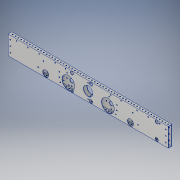
# Autodesk Inventor part: Side Extrusion
Saved by Autodesk Inventor 2019.4 (Build 234330000, 330)
## iProperties
Created: 2019-11-02
Part Number: Side Extrusion
Material: Aluminum 6061
Document SubType Name: Modeling
Designer: admin
Density: 2.7 g/cm^3
Appearance: Aluminum - Flat
Mass: 949.784 g
Surface Area: 3620.83 cm^2
Volume: 351.772 cm^3
Author: admin
Autodesk Inventor part; units mm, degrees
ref_plane "YZ Plane" through (0, 0, 0) normal (1, 0, 0) x (0, 1, 0)
ref_plane "XZ Plane" through (0, 0, 0) normal (0, 1, 0) x (-1, 0, 0)
ref_plane "XY Plane" through (0, 0, 0) normal (0, 0, 1) x (1, 0, 0)
sketch "Sketch1" plane through (0, 0, 0) normal (1, 0, 0) x (0, 1, 0)
  line L0 (-50, 10) -> (50, 10)
  line L1 (50, 10) -> (50, -10)
  line L2 (50, -10) -> (-50, -10)
  line L3 (-50, -10) -> (-50, 10)
  line L4 (-50, 10) -> (50, -10) construction
  line L5 (50, 10) -> (-50, -10) construction
  line L6 (48, -8) -> (48, 8)
  line L7 (48, 8) -> (-48, 8)
  line L8 (-48, 8) -> (-48, -8)
  line L9 (-48, -8) -> (48, -8)
  point P0 (0, 0)
  dimension "d0" = 100
  dimension "d1" = 20
  dimension "d2" = 2
  constraints: 20 end point, 4 parallel, 2 midpoint, 2 perpendicular, 1 horizontal, 3 other
  measures "d0" distance of L1.end L2.end
  measures "d1" distance of L0.end L1.end
  measures "d2" distance between parallel lines of L1 L6
extrude "Extrusion1" add sketch "Sketch1" along normal blind 850
sketch "Sketch2" plane through (0, -50, 10) normal (0, 0, -1) x (-1, 0, 0)
  circle A0 centre (-200, 18.3) radius 16.3
  line L0 (0, 0) -> (-850, 0) projected
  line L1 (0, 100) -> (0, 0) projected
  line L2 (0, 100) -> (-850, 100) projected
  line L3 (0, 0) -> (-850, 0) projected
  circle A1 centre (-650, 18.3) radius 16.3
  line L4 (-850, 100) -> (-850, 0) projected
  point P0 (0, 50)
  dimension "d5" = 32.6
  dimension "d9" = 200
  dimension "d113" = 200
  constraints: 2 centre point
  measures "d5" diameter of A0
  measures "d9" distance from line of L1 A0.centre
  measures "d113" distance from line of L4 A1.centre
extrude "Extrusion2" cut sketch "Sketch2" along normal blind 2 contours A0 | A1
sketch "Sketch3" plane through (0, -50, 10) normal (0, 0, 1) x (1, 0, 0)
  circle A0 centre (320, 36) radius 34
  line L0 (0, 0) -> (0, 100) projected
  line L1 (0, 0) -> (850, 0) projected
  line L2 (425, 100) -> (425, 0)
  circle A1 centre (530, 36) radius 34
  point P0 (0, 50)
  dimension "d10" = 68
  dimension "d11" = 320
  dimension "d12" = 36
  constraints: 2 centre point, 2 end point, 1 midpoint, 1 symmetric about line, 1 other
  measures "d10" diameter of A0
  measures "d11" distance from line of L0 A0.centre
  measures "d12" distance from line of A0.centre L1
extrude "Extrusion3" cut sketch "Sketch3" against normal blind 2
sketch "Sketch4" plane through (0, -50, -10) normal (0, 0, -1) x (-1, 0, 0)
  circle A0 centre (-200, 18.3) radius 16.3 construction
  circle A1 centre (-200, 18.3) radius 16.3 construction
  circle A2 centre (-200, 18.3) radius 12.3
  line L0 (0, 0) -> (-850, 0) projected
  line L1 (-425, 0) -> (-425, 100)
  line L2 (0, 100) -> (-850, 100) projected
  circle A3 centre (-650, 18.3) radius 12.3
  point P0 (0, 50)
  point P1 (-200, 2)
  dimension "d17" = 24.6
  constraints: 2 centre point, 2 end point, 2 midpoint, 1 coincident, 1 symmetric about line, 1 vertical alignment, 1 other
  measures "d17" diameter of A2
extrude "Extrusion4" cut sketch "Sketch4" against normal blind 2
sketch "Sketch5" plane through (0, -50, -10) normal (0, 0, -1) x (-1, 0, 0)
  circle A0 centre (-216, 18.3) radius 2.25
  circle A1 centre (-200, 18.3) radius 12.3 projected
  line L0 (-200, 18.3) -> (-216, 18.3) construction
  circle A2 centre (-200, 34.3) radius 2.25
  circle A3 centre (-184, 18.3) radius 2.25
  line L1 (0, 100) -> (-850, 100) projected
  line L2 (-425, 100) -> (-425, 0)
  line L3 (0, 0) -> (-850, 0) projected
  circle A4 centre (-634, 18.3) radius 2.25
  circle A5 centre (-650, 34.3) radius 2.25
  circle A6 centre (-666, 18.3) radius 2.25
  point P0 (0, 50)
  dimension "d18" = 4.5
  dimension "d21" = 16
  dimension "d24" = 180
  constraints: 6 centre point, 4 end point, 3 symmetric about line, 2 midpoint, 1 horizontal, 8 other
  measures "d18" diameter of A0
  measures "d21" distance of L0.start L0.end
extrude "Extrusion5" cut sketch "Sketch5" against normal blind 2 contours A0 | A2 | A3 | A4 | A5 | A6
sketch "Sketch6" plane through (0, -50, -10) normal (0, 0, -1) x (-1, 0, 0)
  circle A0 centre (-320, 36) radius 10
  line L0 (0, 0) -> (-850, 0)
  line L1 (0, 100) -> (0, 0)
  circle A1 centre (-320, 36) radius 25.4
  circle A2 centre (-320, 61.4) radius 2.75
  circle A3 centre (-345.4, 36) radius 2.75
  circle A4 centre (-320, 10.6) radius 2.75
  circle A5 centre (-294.6, 36) radius 2.75
  line L2 (-253.082685, 23.409359) -> (-232.819395, 42.510891)
  arc A6 (-232.819395, 42.510891) -> (-221.835325, 43.130108) centre (-228.087042, 56.296226) ccw
  line L3 (-221.835325, 43.130108) -> (-214.280231, 31.689157)
  arc A7 (-214.280231, 31.689157) -> (-219.289116, 21.635076) centre (-200.000275, 18.300226) ccw
  line L4 (-219.289116, 21.635076) -> (-250.702863, 18.243714)
  arc A8 (-253.082685, 23.409359) -> (-250.702863, 18.243714) centre (-251.024866, 21.226383) ccw
  line L5 (-211.509077, 53.460841) -> (-194.873767, 53.460841)
  arc A9 (-192.370348, 52.113987) -> (-194.873767, 53.460841) centre (-194.873767, 50.460841) ccw
  line L6 (-192.370348, 52.113987) -> (-179.138449, 32.076445)
  arc A10 (-175.036603, 16.95297) -> (-179.138449, 32.076445) centre (-200.000275, 18.300226) ccw
  arc A11 (-178.032244, 14.114641) -> (-175.036603, 16.95297) centre (-178.032244, 17.114641) ccw
  arc A12 (-180.454865, 17.224322) -> (-178.032244, 14.114641) centre (-177.459399, 17.059432) ccw
  arc A13 (-180.454865, 17.224322) -> (-207.063381, 36.556544) centre (-200.000275, 18.300226) ccw
  arc A14 (-210.571115, 37.588637) -> (-207.063381, 36.556544) centre (-208.145849, 39.354447) ccw
  line L7 (-210.571115, 37.588637) -> (-215.850481, 44.839623)
  arc A15 (-215.927945, 48.259622) -> (-215.850481, 44.839623) centre (-213.425215, 46.605433) ccw
  arc A16 (-215.927945, 48.259622) -> (-214.338886, 51.456924) centre (-228.087042, 56.296226) ccw
  arc A17 (-211.509077, 53.460841) -> (-214.338886, 51.456924) centre (-211.509077, 50.460841) ccw
  line L8 (-284.50186, 40.584929) -> (-284.231798, 32.883294)
  arc A18 (-288.442052, 30.033928) -> (-284.231798, 32.883294) centre (-287.229955, 32.778162) ccw
  line L9 (-288.442052, 30.033928) -> (-290.947932, 31.140747)
  arc A19 (-305.806233, 47.249065) -> (-290.947932, 31.140747) centre (-279.837042, 56.296226) ccw
  arc A20 (-302.97323, 51.236028) -> (-305.806233, 47.249065) centre (-302.97323, 48.236028) ccw
  line L10 (-302.97323, 51.236028) -> (-295.454783, 51.236028)
  arc A21 (-292.788881, 49.61188) -> (-295.454783, 51.236028) centre (-295.454783, 48.236028) ccw
  arc A22 (-292.788881, 49.61188) -> (-286.19197, 43.179614) centre (-279.837042, 56.296226) ccw
  arc A23 (-284.50186, 40.584929) -> (-286.19197, 43.179614) centre (-287.500018, 40.479797) ccw
  arc A24 (-214.732134, -2.522909) -> (-211.723391, 2.623837) centre (-213.520037, 0.221325) ccw
  line L11 (-214.732134, -2.522909) -> (-233.31096, 5.683148)
  arc A25 (-232.524215, 11.397075) -> (-233.31096, 5.683148) centre (-232.098863, 8.427382) ccw
  line L12 (-232.524215, 11.397075) -> (-221.426068, 12.986676)
  arc A26 (-218.209959, 11.117746) -> (-221.426068, 12.986676) centre (-221.000715, 10.016983) ccw
  arc A27 (-218.209959, 11.117746) -> (-211.723391, 2.623837) centre (-200.000275, 18.300226) ccw
  line L13 (-193.453229, -3.079233) -> (-193.473523, -1.544854)
  arc A28 (-192.26411, 0.31878) -> (-193.473523, -1.544854) centre (-191.473698, -1.518405) ccw
  arc A29 (-192.26411, 0.31878) -> (-186.409522, 4.212215) centre (-200.000275, 18.300226) ccw
  arc A30 (-185.020939, 4.772827) -> (-186.409522, 4.212215) centre (-185.020939, 2.772827) ccw
  line L14 (-185.020939, 4.772827) -> (-183.032662, 4.772827)
  arc A31 (-181.557218, 1.422618) -> (-183.032662, 4.772827) centre (-183.032662, 2.772827) ccw
  arc A32 (-190.710198, -4.909567) -> (-181.557218, 1.422618) centre (-200.000275, 18.300226) ccw
  arc A33 (-193.453229, -3.079233) -> (-190.710198, -4.909567) centre (-191.453404, -3.052783) ccw
  line L15 (-284.569395, 79.544037) -> (-284.569395, 72.078853)
  arc A34 (-286.249506, 69.384806) -> (-284.569395, 72.078853) centre (-287.569395, 72.078853) ccw
  arc A35 (-286.249506, 69.384806) -> (-292.788881, 62.980572) centre (-279.837042, 56.296226) ccw
  arc A36 (-295.454783, 61.356424) -> (-292.788881, 62.980572) centre (-295.454783, 64.356424) ccw
  line L16 (-295.454783, 61.356424) -> (-302.97323, 61.356424)
  arc A37 (-305.806233, 65.343387) -> (-302.97323, 61.356424) centre (-302.97323, 64.356424) ccw
  arc A38 (-288.516214, 82.390707) -> (-305.806233, 65.343387) centre (-279.837042, 56.296226) ccw
  arc A39 (-284.569395, 79.544037) -> (-288.516214, 82.390707) centre (-287.569395, 79.544037) ccw
  line L17 (-228.57644, 83.796226) -> (-228.087042, 83.796226)
  arc A40 (-205.139033, 71.450067) -> (-228.087042, 83.796226) centre (-228.087042, 56.296226) ccw
  line L18 (-205.139033, 71.450067) -> (-200.077204, 63.784757)
  arc A41 (-202.580623, 59.131611) -> (-200.077204, 63.784757) centre (-202.580623, 62.131611) ccw
  line L19 (-202.580623, 59.131611) -> (-211.509077, 59.131611)
  arc A42 (-214.338886, 61.135528) -> (-211.509077, 59.131611) centre (-211.509077, 62.131611) ccw
  arc A43 (-214.338886, 61.135528) -> (-226.317651, 70.763426) centre (-228.087042, 56.296226) ccw
  arc A44 (-228.765396, 72.69578) -> (-226.317651, 70.763426) centre (-225.953454, 73.741237) ccw
  line L20 (-228.765396, 72.69578) -> (-231.388383, 79.750769)
  arc A45 (-228.57644, 83.796226) -> (-231.388383, 79.750769) centre (-228.57644, 80.796226) ccw
  line L21 (-265.77495, 52.463707) -> (-242.149133, 52.463707)
  arc A46 (-242.149133, 52.463707) -> (-238.347574, 45.944796) centre (-228.087042, 56.296226) ccw
  line L22 (-238.347574, 45.944796) -> (-267.246983, 24.918347)
  arc A47 (-271.92876, 26.642518) -> (-267.246983, 24.918347) centre (-269.011975, 27.344208) ccw
  line L23 (-271.92876, 26.642518) -> (-275.089001, 39.779003)
  arc A48 (-273.480579, 43.180357) -> (-275.089001, 39.779003) centre (-272.172217, 40.480693) ccw
  arc A49 (-273.480579, 43.180357) -> (-265.77495, 52.463707) centre (-279.837042, 56.296226) ccw
  line L24 (-244.279549, 60.128745) -> (-263.644534, 60.128745)
  arc A50 (-266.408547, 61.962454) -> (-263.644534, 60.128745) centre (-263.644534, 63.128745) ccw
  arc A51 (-266.408547, 61.962454) -> (-271.422142, 68.196649) centre (-279.837042, 56.296226) ccw
  arc A52 (-272.690087, 70.646136) -> (-271.422142, 68.196649) centre (-269.690087, 70.646136) ccw
  line L25 (-272.690087, 70.646136) -> (-272.690087, 80.796226)
  arc A53 (-269.690087, 83.796226) -> (-272.690087, 80.796226) centre (-269.690087, 80.796226) ccw
  line L26 (-269.690087, 83.796226) -> (-241.990418, 83.796226)
  arc A54 (-239.348489, 82.217567) -> (-241.990418, 83.796226) centre (-241.990418, 80.796226) ccw
  line L27 (-239.348489, 82.217567) -> (-234.326691, 72.883258)
  arc A55 (-235.452561, 68.873179) -> (-234.326691, 72.883258) centre (-236.96862, 71.461917) ccw
  arc A56 (-235.452561, 68.873179) -> (-241.515537, 61.962454) centre (-228.087042, 56.296226) ccw
  arc A57 (-244.279549, 60.128745) -> (-241.515537, 61.962454) centre (-244.279549, 63.128745) ccw
  circle A58 centre (-188.087042, 69.219) radius 2.75
  circle A59 centre (-277.837042, 16.582759) radius 2.75
  circle A60 centre (-250.087042, 92.776017) radius 2.75
  circle A61 centre (-160.000305, 27.300362) radius 2.75
  circle A62 centre (-313.422276, 79.81286) radius 2.75
  circle A63 centre (-200.000275, 18.300226) radius 9.575
  circle A64 centre (-228.087042, 56.296226) radius 9.575
  circle A65 centre (-279.837042, 56.296226) radius 9.575
  arc A66 (-244.094047, 93.065872) -> (-256.080036, 92.486162) centre (-250.087042, 92.776017) ccw
  line L28 (-256.080036, 92.486162) -> (-281.527863, 91.255361)
  arc A67 (-281.527863, 91.255361) -> (-302.063851, 83.332663) centre (-279.837042, 56.296226) ccw
  line L29 (-312.063851, 85.657061) -> (-302.063851, 83.332663)
  arc A68 (-312.063851, 85.657061) -> (-318.449419, 76.537524) centre (-313.422276, 79.81286) ccw
  line L30 (-312.844999, 67.935588) -> (-318.449419, 76.537524)
  arc A69 (-312.844999, 67.935588) -> (-294.877776, 24.692804) centre (-279.837042, 56.296226) ccw
  line L31 (-294.877776, 24.692804) -> (-283.254771, 19.16117)
  arc A70 (-283.254771, 19.16117) -> (-272.419312, 14.004347) centre (-277.837042, 16.582759) ccw
  line L32 (-272.419312, 14.004347) -> (-215.041009, -13.303196)
  arc A71 (-169.897664, 36.156116) -> (-170.793719, 37.586933) centre (-200.000275, 18.300226) ccw
  line L33 (-160.000305, 21.300362) -> (-162.000275, 21.300362)
  arc A72 (-160.000305, 21.300362) -> (-156.580779, 22.370166) centre (-160.000305, 27.300362) ccw
  arc A73 (-215.041009, -13.303196) -> (-165.000275, 18.300352) centre (-200.000275, 18.300226) ccw
  line L34 (-170.793719, 37.586933) -> (-184.354376, 58.122326)
  arc A74 (-187.633238, 75.201814) -> (-191.393334, 74.225838) centre (-188.087042, 69.219) ccw
  line L35 (-195.5499, 75.076111) -> (-196.794303, 76.960555)
  arc A75 (-196.794303, 76.960555) -> (-229.898636, 93.752442) centre (-228.087042, 56.296226) ccw
  line L36 (-229.898636, 93.752442) -> (-244.094047, 93.065872)
  line L37 (0, 100) -> (-850, 100)
  line L38 (-425, 100) -> (-425, 0)
  circle A76 centre (-530, 61.4) radius 2.75
  circle A77 centre (-504.6, 36) radius 2.75
  circle A78 centre (-530, 10.6) radius 2.75
  circle A79 centre (-555.4, 36) radius 2.75
  circle A80 centre (-661.912958, 69.219) radius 2.75
  circle A81 centre (-572.162958, 16.582759) radius 2.75
  circle A82 centre (-599.912958, 92.776017) radius 2.75
  circle A83 centre (-689.999695, 27.300362) radius 2.75
  circle A84 centre (-536.577724, 79.81286) radius 2.75
  line L39 (-156.580779, 22.370166) -> (-137.281762, 35.755737)
  arc A85 (-137.281762, 35.755737) -> (-147.167505, 72.132439) centre (-148.680183, 52.189726) ccw
  line L40 (-147.167505, 72.132439) -> (-187.633238, 75.201814)
  arc A86 (-195.5499, 75.076111) -> (-191.393334, 74.225838) centre (-193.046481, 76.729257) ccw
  arc A87 (-162.000275, 21.300362) -> (-165.000275, 18.300352) centre (-162.000275, 18.300362) ccw
  circle A88 centre (-148.680183, 52.189726) radius 10.5
  circle A89 centre (-163.234444, 48.560195) radius 1.65
  arc A90 (-181.624055, 62.766879) -> (-184.354376, 58.122326) centre (-181.850957, 59.775472) ccw
  line L41 (-181.624055, 62.766879) -> (-170.444252, 61.918877)
  arc A91 (-167.802767, 58.048634) -> (-170.444252, 61.918877) centre (-170.671154, 58.92747) ccw
  arc A92 (-167.802767, 58.048634) -> (-164.446092, 39.883788) centre (-148.680183, 52.189726) ccw
  arc A93 (-165.101215, 35.572799) -> (-164.446092, 39.883788) centre (-166.810978, 38.037897) ccw
  line L42 (-165.101215, 35.572799) -> (-165.607677, 35.221523)
  arc A94 (-169.897664, 36.156116) -> (-165.607677, 35.221523) centre (-167.31744, 37.686621) ccw
  circle A95 centre (-144.546319, 66.608851) radius 1.65
  circle A96 centre (-138.259787, 41.400132) radius 1.65
  circle A97 centre (-530, 36) radius 10
  point P0 (0, 50)
  point P1 (-200.000275, 18.300226)
  point P2 (-200.000275, 18.300226)
  dimension "d31" = 50.8
  dimension "d28" = 20
  dimension "d29" = 36
  dimension "d30" = 320
  dimension "d32" = 5.5
  dimension "d35" = 360
  dimension "d46" = 36
  constraints: 15 centre point, 10 symmetric about line, 2 end point, 2 midpoint, 1 coincident, 1 vertical alignment, 21 other
  measures "d28" diameter of A0
  measures "d29" distance from line of L0 A0.centre
  measures "d30" distance from line of L1 A0.centre
  measures "d32" diameter of A2
  measures "d46" distance from line of L0 A3.centre
extrude "Extrusion6" cut sketch "Sketch6" against normal blind 50 contours A0 | A2 A1 | A1 A2 | A4 A1 | A1 A4 | A5 A1 | A1 A5 A19 | A5 A19 | A3 A1 | A1 A3 | A58 | A59 | A60 | A61 | A62 | A76 | A77 | A78 | A79 | A80 | A81 | A82 | A83 | A84 | A97 picked at (-296.100043, 35.292407)
sketch "Sketch7" plane through (0, -50, -10) normal (0, 0, -1) x (-1, 0, 0)
  circle A0 centre (-228.087, 56.296) radius 10.5
  line L0 (0, 100) -> (-850, 100) projected
  line L1 (0, 100) -> (0, 0) projected
  circle A1 centre (-279.787, 56.296) radius 10.5
  line L2 (-228.087, 56.296) -> (-279.787, 56.296) construction
  line L3 (-425, 100) -> (-425, 0)
  circle A2 centre (-621.913, 56.296) radius 10.5
  circle A3 centre (-570.213, 56.296) radius 10.5
  point P0 (0, 50)
  dimension "d39" = 43.704
  dimension "d40" = 228.087
  dimension "d41" = 21
  dimension "d44" = 21
  dimension "d45" = 51.7
  constraints: 4 centre point, 4 end point, 2 symmetric about line, 1 horizontal, 1 midpoint, 1 vertical, 2 other
  measures "d39" distance from line of L0 L2.start
  measures "d40" distance from line of L1 L2.start
  measures "d41" diameter of A0
  measures "d44" diameter of A1
  measures "d45" distance of L2.start L2.end
extrude "Extrusion7" cut sketch "Sketch7" against normal up to surface (2 mm away)
sketch "Sketch8" plane through (0, -50, -10) normal (0, 0, -1) x (-1, 0, 0)
  circle A0 centre (-425, 87.5) radius 2.75
  circle A1 centre (-545, 92) radius 2.75
  circle A2 centre (-685, 90.5) radius 2.75
  circle A3 centre (-805, 90.5) radius 2.75
  circle A4 centre (-745, 90.5) radius 2.75
  circle A5 centre (-837.5, 50) radius 2.75
  circle A6 centre (-837.5, 80) radius 2.75
  circle A7 centre (-837.5, 20) radius 2.75
  circle A8 centre (-425, 12.5) radius 2.75
  circle A9 centre (-545, 8) radius 2.75
  line L0 (-850, 0) -> (-850, 100) construction
  line L1 (0, 100) -> (-850, 100) construction
  line L2 (0, 0) -> (-850, 0) construction
  line L3 (0, 0) -> (-850, 0) construction
  line L4 (-425, 0) -> (-425, 100)
  circle A10 centre (-305, 92) radius 2.75
  circle A11 centre (-165, 90.5) radius 2.75
  circle A12 centre (-45, 90.5) radius 2.75
  circle A13 centre (-105, 90.5) radius 2.75
  circle A14 centre (-12.5, 50) radius 2.75
  circle A15 centre (-12.5, 80) radius 2.75
  circle A16 centre (-12.5, 20) radius 2.75
  circle A17 centre (-305, 8) radius 2.75
  line L5 (0, 0) -> (0, 100) construction
  line L6 (0, 0) -> (-850, 0) construction
  line L7 (0, 0) -> (-850, 0) projected
  line L8 (0, 100) -> (0, 0) projected
  line L9 (-850, 0) -> (-850, 100) projected
  dimension "d49" = 5.5
  dimension "d50" = 5.5
  dimension "d51" = 5.5
  dimension "d52" = 12.5
  dimension "d53" = 12.5
  dimension "d54" = 12.5
  dimension "d55" = 20
  dimension "d56" = 20
  dimension "d57" = 50
  dimension "d58" = 45
  dimension "d59" = 105
  dimension "d60" = 60
  dimension "d61" = 9.5
  dimension "d62" = 9.5
  dimension "d63" = 9.5
  dimension "d64" = 5.5
  dimension "d65" = 5.5
  dimension "d66" = 5.5
  dimension "d80" = 12.5
  dimension "d81" = 8
  dimension "d84" = 8
  dimension "d88" = 305
  dimension "d89" = 305
  dimension "d90" = 12.5
  dimension "d91" = 100
  dimension "d133" = 90
  constraints: 18 centre point, 14 end point, 8 symmetric about line, 4 equal radius, 3 collinear, 3 point on line, 2 midpoint, 8 other
  measures "d49" diameter of A6
  measures "d50" diameter of A5
  measures "d51" diameter of A7
  measures "d52" distance from line of L0 A7.centre
  measures "d53" distance from line of L0 A5.centre
  measures "d54" distance from line of L0 A6.centre
  measures "d55" distance from line of L1 A6.centre
  measures "d56" distance from line of L2 A7.centre
  measures "d57" distance from line of L1 A5.centre
  measures "d58" distance from line of L0 A3.centre
  measures "d59" distance from line of L0 A4.centre
  measures "d60" distance of A4.centre A2.centre
  measures "d61" distance from line of L1 A3.centre
  measures "d62" distance from line of L1 A4.centre
  measures "d63" distance from line of L1 A2.centre
  measures "d64" diameter of A3
  measures "d65" diameter of A4
  measures "d66" diameter of A2
  measures "d80" distance from line of L2 A8.centre
  measures "d81" distance from line of L2 A9.centre
  measures "d84" distance from line of L1 A1.centre
  measures "d88" distance from line of L0 A1.centre
  measures "d89" distance from line of L0 A9.centre
  measures "d90" distance from line of L1 A0.centre
  measures "d91" distance between parallel lines of L1 L3
  measures "d133" angle of L1 L5
extrude "Extrusion8" cut sketch "Sketch8" against normal blind 50
sketch "Sketch9" plane through (0, -50, 10) normal (0, 0, 1) x (1, 0, 0)
  circle A0 centre (272.5, 62.5) radius 2.75
  circle A1 centre (272.5, 37.5) radius 2.75
  line L0 (0, 100) -> (850, 100) projected
  line L1 (425, 100) -> (425, 0)
  line L2 (0, 0) -> (850, 0) projected
  line L3 (0, 0) -> (0, 100) projected
  circle A2 centre (577.5, 62.5) radius 2.75
  circle A3 centre (577.5, 37.5) radius 2.75
  point P0 (0, 50)
  dimension "d94" = 5.5
  dimension "d95" = 5.5
  dimension "d96" = 272.5
  dimension "d97" = 272.5
  dimension "d98" = 37.5
  dimension "d99" = 37.5
  constraints: 4 centre point, 2 end point, 2 midpoint, 2 symmetric about line, 2 other
  measures "d94" diameter of A0
  measures "d95" diameter of A1
  measures "d96" distance from line of L3 A0.centre
  measures "d97" distance from line of L3 A1.centre
  measures "d98" distance from line of L2 A1.centre
  measures "d99" distance from line of L0 A0.centre
extrude "Extrusion9" cut sketch "Sketch9" against normal blind 5 contours A0 | A1 | A2 | A3
sketch "Sketch10" plane through (0, 50, 10) normal (0, 1, 0) x (1, 0, 0)
  line L0 (0, 20) -> (850, 20) projected
  circle A0 centre (15, 10) radius 2.75
  line L1 (15, 10) -> (0, 10) construction
  circle A1 centre (30, 10) radius 2.75
  circle A2 centre (45, 10) radius 2.75
  circle A3 centre (60, 10) radius 2.75
  circle A4 centre (75, 10) radius 2.75
  circle A5 centre (90, 10) radius 2.75
  circle A6 centre (105, 10) radius 2.75
  circle A7 centre (120, 10) radius 2.75
  circle A8 centre (135, 10) radius 2.75
  circle A9 centre (150, 10) radius 2.75
  circle A10 centre (165, 10) radius 2.75
  circle A11 centre (180, 10) radius 2.75
  circle A12 centre (195, 10) radius 2.75
  circle A13 centre (210, 10) radius 2.75
  circle A14 centre (225, 10) radius 2.75
  circle A15 centre (240, 10) radius 2.75
  circle A16 centre (255, 10) radius 2.75
  circle A17 centre (270, 10) radius 2.75
  circle A18 centre (285, 10) radius 2.75
  circle A19 centre (300, 10) radius 2.75
  circle A20 centre (315, 10) radius 2.75
  circle A21 centre (330, 10) radius 2.75
  circle A22 centre (345, 10) radius 2.75
  circle A23 centre (360, 10) radius 2.75
  circle A24 centre (375, 10) radius 2.75
  circle A25 centre (390, 10) radius 2.75
  circle A26 centre (405, 10) radius 2.75
  circle A27 centre (420, 10) radius 2.75
  circle A28 centre (435, 10) radius 2.75
  circle A29 centre (450, 10) radius 2.75
  circle A30 centre (465, 10) radius 2.75
  circle A31 centre (480, 10) radius 2.75
  circle A32 centre (495, 10) radius 2.75
  circle A33 centre (510, 10) radius 2.75
  circle A34 centre (525, 10) radius 2.75
  circle A35 centre (540, 10) radius 2.75
  circle A36 centre (555, 10) radius 2.75
  circle A37 centre (570, 10) radius 2.75
  circle A38 centre (585, 10) radius 2.75
  circle A39 centre (600, 10) radius 2.75
  circle A40 centre (615, 10) radius 2.75
  circle A41 centre (630, 10) radius 2.75
  circle A42 centre (645, 10) radius 2.75
  circle A43 centre (660, 10) radius 2.75
  circle A44 centre (675, 10) radius 2.75
  circle A45 centre (690, 10) radius 2.75
  circle A46 centre (705, 10) radius 2.75
  circle A47 centre (720, 10) radius 2.75
  circle A48 centre (735, 10) radius 2.75
  circle A49 centre (750, 10) radius 2.75
  circle A50 centre (765, 10) radius 2.75
  circle A51 centre (780, 10) radius 2.75
  circle A52 centre (795, 10) radius 2.75
  circle A53 centre (810, 10) radius 2.75
  circle A54 centre (825, 10) radius 2.75
  circle A55 centre (840, 10) radius 2.75
  dimension "d102" = 5.5
  dimension "d103" = 15
  dimension "d106" = 15
  constraints: 56 centre point, 2 end point, 2 horizontal, 110 other
  measures "d102" diameter of A0
  measures "d103" distance of L1.start L1.end
  measures "d106" distance of L1.start A1.centre
extrude "Extrusion10" cut sketch "Sketch10" against normal through all
sketch "Sketch11" plane through (0, -50, -10) normal (0, 0, -1) x (-1, 0, 0)
  point P0 (0, 50)
sketch "Sketch12" plane through (0, -50, -10) normal (0, 0, -1) x (-1, 0, 0)
  circle A0 centre (-577.5, 62.5) radius 2.75 projected
  circle A1 centre (-577.5, 62.5) radius 2.75 projected
  circle A2 centre (-577.5, 37.5) radius 2.75 projected
  circle A3 centre (-577.5, 37.5) radius 2.75 projected
  circle A4 centre (-272.5, 62.5) radius 2.75 projected
  circle A5 centre (-272.5, 62.5) radius 2.75 projected
  circle A6 centre (-272.5, 37.5) radius 2.75 projected
  circle A7 centre (-272.5, 37.5) radius 2.75 projected
  circle A8 centre (-577.5, 37.5) radius 7.5
  circle A9 centre (-272.5, 37.5) radius 7.5
  point P0 (0, 50)
  dimension "d114" = 15
  dimension "d115" = 15
  constraints: 2 centre point, 2 coincident
  measures "d114" diameter of A8
  measures "d115" diameter of A9
extrude "Extrusion11" cut sketch "Sketch12" against normal blind 2 contours A2 | A6 | A8 | A9
sketch "Sketch13" plane through (0, -50, -10) normal (0, 0, -1) x (-1, 0, 0)
  circle A0 centre (-789.4, 90) radius 2.75 projected
  circle A1 centre (-789.5, 10) radius 2.75 projected
  circle A2 centre (-440.6, 90) radius 2.75 projected
  circle A3 centre (-440.6, 10) radius 2.75 projected
  circle A4 centre (-339.4, 90) radius 2.75 projected
  circle A5 centre (-339.4, 10) radius 2.75 projected
  point P0 (0, 50)
extrude "Extrusion12" cut sketch "Sketch13" against normal through all
sketch "Sketch14" plane through (0, -50, 10) normal (0, 0, 1) x (1, 0, 0)
  circle A0 centre (339.4, 90) radius 2.75
  circle A1 centre (789.4, 90) radius 2.75
  circle A2 centre (789.5, 10) radius 2.75
  circle A3 centre (440.6, 10) radius 2.75
  circle A4 centre (440.6, 90) radius 2.75
  circle A5 centre (339.4, 90) radius 2.75
  circle A6 centre (339.4, 10) radius 2.75
  circle A7 centre (339.4, 90) radius 8.75
  circle A8 centre (339.4, 10) radius 8.75
  circle A9 centre (440.6, 10) radius 8.75
  circle A10 centre (440.6, 90) radius 8.75
  circle A11 centre (789.4, 90) radius 8.75
  circle A12 centre (789.5, 10) radius 8.75
  point P0 (0, 50)
extrude "Extrusion13" cut sketch "Sketch14" against normal blind 3
sketch "Sketch15" plane through (0, -50, -10) normal (0, 0, -1) x (-1, 0, 0)
  circle A0 centre (-425, 50) radius 25
  line L0 (0, 0) -> (-850, 0) projected
  line L1 (0, 100) -> (0, 0) projected
  point P0 (0, 50)
  dimension "d128" = 50
  dimension "d129" = 50
  dimension "d130" = 425
  constraints: 1 centre point
  measures "d128" diameter of A0
  measures "d129" distance from line of L0 A0.centre
  measures "d130" distance from line of L1 A0.centre
extrude "Extrusion14" cut sketch "Sketch15" against normal blind 65.5
sketch "Sketch16" plane through (0, -50, -10) normal (0, 0, -1) x (-1, 0, 0)
  circle A0 centre (-425, 12.5) radius 2.75 projected
  circle A1 centre (-425, 12.5) radius 7.75
  point P0 (0, 50)
  dimension "d134" = 5
  constraints: 1 centre point
  measures "d134" radial gap between concentric circles of A0 A1
extrude "Extrusion15" cut sketch "Sketch16" against normal blind 2
sketch "Sketch17" plane through (0, -50, -10) normal (0, 0, -1) x (-1, 0, 0)
  circle A0 centre (-805, 90.5) radius 2.75 projected
  circle A1 centre (-805, 90.5) radius 6.75
  point P0 (0, 50)
  dimension "d137" = 4
  constraints: 1 centre point
  measures "d137" radial gap between concentric circles of A0 A1
extrude "Extrusion16" cut sketch "Sketch17" against normal blind 2
equation "\"d97\" = d96"
equation "\"d98\" = d99"
body "Solid1"
